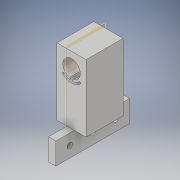
# Autodesk Inventor part: AxleBracket
Saved by Autodesk Inventor 2018 (Build 220112000, 112)
## iProperties
Created: 2019-02-07
Part Number: AxleBracket
Material: Generic
Document SubType Name: Modeling
Designer: anirudh
Density: 1 g/cm^3
Appearance: Default
Author: anirudh
Autodesk Inventor part; units mm, degrees
ref_plane "YZ Plane" through (0, 0, 0) normal (1, 0, 0) x (0, 1, 0)
ref_plane "XZ Plane" through (0, 0, 0) normal (0, 1, 0) x (-1, 0, 0)
ref_plane "XY Plane" through (0, 0, 0) normal (0, 0, 1) x (1, 0, 0)
sketch "Sketch1" plane through (0, 0, 0) normal (1, 0, 0) x (0, 1, 0)
  line L0 (0, 0) -> (35.814, 0)
  line L1 (35.814, 0) -> (35.814, -25.4)
  line L2 (35.814, -25.4) -> (0, -25.4)
  line L3 (0, -25.4) -> (0, 0)
  constraints: 8 end point, 2 parallel, 1 horizontal, 1 perpendicular
extrude "Extrusion1" add sketch "Sketch1" along normal blind 15
ref_plane "Work Plane1" through (0, 5.08, -25.4) normal (0, 1, 0) x (1, 0, 0)
sketch "Sketch5" plane through (0, 35.814, 0) normal (0, 0, 1) x (1, 0, 0)
  line L0 (0, 0) -> (15, 0) projected
  line L1 (0, 0) -> (15, 0)
  line L2 (15, 0) -> (15, 12.7)
  line L3 (15, 12.7) -> (0, 12.7)
  line L4 (0, 12.7) -> (0, 0)
  point P0 (0, -35.814)
  dimension "d13" = 12.7
  constraints: 8 end point, 2 parallel, 1 horizontal, 1 perpendicular
  measures "d13" distance of L2.end L1.end
extrude "Extrusion5" add sketch "Sketch5" against normal blind 25.4
ref_plane "Work Plane2" through (0, 5.08, 0) normal (0, 0, 1) x (1, 0, 0)
sketch "Sketch6" plane through (0, 5.08, 0) normal (0, 0, 1) x (1, 0, 0)
  line L0 (0, 0) -> (0, 43.434) projected
  line L1 (15, 0) -> (15, 43.434) projected
  arc A0 (8.785, 27.2013) -> (6.2434, 27.1951) centre (7.5, 33.0621) ccw
  arc A1 (8.785, 27.2013) -> (6.2434, 27.1951) centre (7.5, 33.0621) ccw
  arc A2 (1.4653, 27.0273) -> (13.5347, 27.0273) centre (7.5, 33.0621) ccw
  arc A3 (5.9165, 25.9724) -> (6.2434, 27.1951) centre (6.0079, 26.603) ccw
  arc A4 (5.8135, 25.9962) -> (6.056, 27.2384) centre (6.0079, 26.603) ccw
  arc A5 (8.785, 27.2013) -> (9.0971, 25.9754) centre (8.8835, 26.5737) ccw
  arc A6 (8.785, 27.2013) -> (9.0971, 25.9754) centre (8.8835, 26.5737) ccw
  arc A7 (2.3633, 27.9254) -> (1.4653, 27.0273) centre (1.9143, 27.4764) ccw
  arc A8 (2.3633, 27.9254) -> (1.4653, 27.0273) centre (1.9143, 27.4764) ccw
  arc A9 (13.5347, 27.0273) -> (12.6367, 27.9254) centre (13.0857, 27.4764) ccw
  arc A10 (13.5347, 27.0273) -> (12.6367, 27.9254) centre (13.0857, 27.4764) ccw
  arc A11 (2.3633, 27.9254) -> (5.9165, 25.9724) centre (7.5, 33.0621) ccw
  arc A12 (9.0971, 25.9754) -> (12.6367, 27.9254) centre (7.5, 33.0621) ccw
  point P0 (0, -5.08)
  constraints: 34 point on circle, 13 centre point, 7 coincident
sketch "Sketch7" plane through (15, 0, 0) normal (1, 0, 0) x (0, 0, -1)
  line L0 (0, 0) -> (0, 48.514) projected
  line L1 (0, 48.514) -> (25.4, 48.514)
  line L2 (25.4, 48.514) -> (25.4, 5.08)
  line L3 (25.4, 0) -> (0, 0)
  line L4 (0, 5.08) -> (0, 48.514)
  line L5 (-15, 5.08) -> (-15, 0) projected
  line L6 (25.4, 0) -> (25.4, 0) projected
  line L7 (40.4, 5.08) -> (40.4, 0)
  line L8 (40.4, 0) -> (-15, 0)
  line L9 (-15, 0) -> (-15, 5.08)
  line L10 (-15, 5.08) -> (0, 5.08)
  line L11 (25.4, 5.08) -> (40.4, 5.08)
  point P0 (0, 5.08)
  constraints: 18 end point, 5 parallel, 3 horizontal, 3 perpendicular, 1 other
extrude "Extrusion6" add sketch "Sketch7" along normal blind 2.54
sketch "Sketch8" plane through (0, 0, 0) normal (-1, 0, 0) x (0, 0, 1)
  line L0 (-40.4, 0) -> (-40.4, 5.08) projected
  line L1 (-40.4, 0) -> (0, 0) projected
  line L2 (15, 5.08) -> (15, 0)
  line L3 (15, 0) -> (-40.4, 0)
  line L4 (-40.4, 0) -> (-40.4, 5.08)
  line L5 (-25.4, 48.514) -> (-25.4, 0) projected
  line L6 (-25.4, 48.514) -> (0, 48.514)
  line L7 (0, 48.514) -> (0, 5.08)
  line L8 (0, 0) -> (-25.4, 0)
  line L9 (-25.4, 5.08) -> (-25.4, 48.514)
  line L10 (-40.4, 5.08) -> (-25.4, 5.08)
  line L11 (0, 5.08) -> (15, 5.08)
  constraints: 18 end point, 5 parallel, 3 horizontal, 3 perpendicular
extrude "Extrusion7" add sketch "Sketch8" along normal blind 2.54
extrude "Extrusion8" cut sketch "Sketch6" against normal blind 57.785
sketch "Sketch9" plane through (0, 5.08, 15) normal (0, 1, 0) x (1, 0, 0)
  line L0 (-2.54, 55.4) -> (-2.54, 0) projected
  line L1 (17.54, 15) -> (17.54, 0) projected
  line L2 (-2.54, 0) -> (17.54, 0)
  line L3 (17.54, 0) -> (17.54, 15)
  line L4 (17.54, 15) -> (-2.54, 15)
  line L5 (-2.54, 15) -> (-2.54, 0)
  line L6 (0, 55.4) -> (-2.54, 55.4) projected
  line L7 (17.54, 55.4) -> (17.54, 40.4) projected
  line L8 (-2.54, 55.4) -> (17.54, 55.4)
  line L9 (17.54, 55.4) -> (17.54, 40.4)
  line L10 (17.54, 40.4) -> (-2.54, 40.4)
  line L11 (-2.54, 40.4) -> (-2.54, 55.4)
  point P0 (0, 15)
  constraints: 16 end point, 4 parallel, 2 horizontal, 2 perpendicular
extrude "Extrusion9" cut sketch "Sketch9" against normal blind 57.785
sketch "Sketch10" plane through (17.54, 0, -25.4) normal (0, -1, 0) x (1, 0, 0)
  line L0 (-20.08, 0) -> (-20.08, 25.4) projected
  line L1 (-20.08, 0) -> (0, 0) projected
  line L2 (-20.08, 25.4) -> (0, 25.4)
  line L3 (0, 25.4) -> (0, 0)
  line L4 (0, 0) -> (-20.08, 0)
  line L5 (-20.08, 0) -> (-20.08, 25.4)
  point P0 (-17.54, 25.4)
  constraints: 8 end point, 2 parallel, 1 horizontal, 1 perpendicular
extrude "Extrusion10" cut sketch "Sketch10" against normal blind 2.3368
ref_plane "Work Plane3" through (4.332, 0, 0) normal (1, 0, 0) x (0, 0, -1)
sketch "Sketch11" plane through (4.332, 0, 0) normal (1, 0, 0) x (0, 0, -1)
  line L0 (0, 2.3368) -> (0, 48.514) projected
  line L1 (0, 2.3368) -> (-12.7, 2.3368)
  line L2 (25.4, 2.3368) -> (0, 2.3368) projected
  line L3 (25.4, 2.3368) -> (38.1, 2.3368)
  line L4 (-12.7, 2.3368) -> (38.1, 2.3368)
  line L5 (38.1, 2.3368) -> (38.1, -12.6632)
  line L6 (38.1, -12.6632) -> (-12.7, -12.6632)
  line L7 (-12.7, -12.6632) -> (-12.7, 2.3368)
  circle A0 centre (12.7, -5.1632) radius 1.85
  circle A1 centre (-3.175, -5.1632) radius 1.85
  circle A2 centre (28.575, -5.1632) radius 1.85
  point P0 (0, 0)
  dimension "d28" = 12.7
  dimension "d29" = 12.7
  dimension "d30" = 15
  dimension "d32" = 3.7
  dimension "d35" = 3.7
  dimension "d36" = 3.7
  constraints: 12 end point, 3 centre point, 3 horizontal, 2 parallel, 1 perpendicular
  measures "d28" distance of L0.start L1.end
  measures "d29" distance of L2.start L3.end
  measures "d30" distance of L4.end L5.end
  measures "d32" diameter of A0
  measures "d35" diameter of A1
  measures "d36" diameter of A2
extrude "Extrusion11" add sketch "Sketch11" along normal blind 5.08
body "Solid1"
